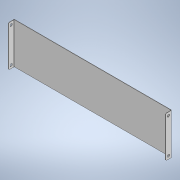
# Autodesk Inventor part: Conector
Saved by Autodesk Inventor 2021.2 (Build 252289000, 289)
## iProperties
Created: 2026-06-03
Part Number: Conector
Material: Generic
Document SubType Name: Sheet Metal
Designer: NELSON
Density: 1 g/cm^3
Sheet Metal Rule: Por defecto_mm
Appearance: Default
Author: NELSON
Autodesk Inventor part; units mm, degrees
ref_plane "YZ Plane" through (0, 0, 0) normal (1, 0, 0) x (0, 1, 0)
ref_plane "XZ Plane" through (0, 0, 0) normal (0, 1, 0) x (-1, 0, 0)
ref_plane "XY Plane" through (0, 0, 0) normal (0, 0, 1) x (1, 0, 0)
sketch "Boceto1" plane through (0, 0, 0) normal (0, 0, 1) x (1, 0, 0)
  line L0 (386.3, -100) -> (-386.3, -100)
  line L1 (-386.3, -100) -> (-386.3, 100)
  line L2 (-386.3, 100) -> (386.3, 100)
  line L3 (386.3, 100) -> (386.3, -100)
  line L4 (386.3, -100) -> (-386.3, 100) construction
  line L5 (-386.3, -100) -> (386.3, 100) construction
  point P0 (0, 0)
  dimension "d0" = 772.6
  dimension "d1" = 200
  measures "d0" distance of L1.end L2.end
  measures "d1" distance of L2.end L0.start
extrude "Placa1" add sketch "Boceto1" along normal blind 2
sketch "Boceto2" plane through (-384.3, -100, 0) normal (-1, 0, 0) x (0, -1, 0)
  line L0 (-200, 0) -> (0, 0)
  line L1 (0, 0) -> (0, 30)
  line L2 (0, 30) -> (-200, 30)
  line L3 (-200, 30) -> (-200, 0)
  constraints: 6 end point, 1 horizontal, 1 perpendicular, 1 vertical
edge flange "Pestaña1" height 30 angle 90 thickness 2 bend radius 2 thickness toward (-1, 0, 0) relief tear relief width 2 relief depth 1 corner gap 2 corner form 0 edges at (-386.3, 0, 2) (386.3, 0, 2) wall of the first edge with corners at (-384.3, 100, 0) (-384.3, -100, 0) (-384.3, -100, 30) (-384.3, 100, 30)
bend "Doblez1"
corner "Esquina1"
sketch "Boceto3" plane through (386.3, -100, 30) normal (1, 0, 0) x (0, 0, -1)
  circle A0 centre (13, 185) radius 6
  circle A1 centre (13, 15) radius 6
  line L0 (26, 0) -> (0, 0) projected
  line L1 (0, 200) -> (26, 200) projected
  point P0 (30, 100)
  point P1 (13, 0)
  point P2 (13, 200)
  dimension "d13" = 12
  dimension "d14" = 12
  dimension "d16" = 15
  dimension "d17" = 15
  constraints: 2 centre point, 2 midpoint, 2 vertical alignment
  measures "d13" diameter of A0
  measures "d14" diameter of A1
  measures "d16" distance from line of L0 A1.centre
  measures "d17" distance from line of A0.centre L1
extrude "Extrusión1" cut sketch "Boceto3" against normal through all
fillet "Redondeo de esquina1" radius 6 4 edges at (385.3, -100, 30) (-385.3, -100, 30) (-385.3, 100, 30) (385.3, 100, 30)
equation "\"d2\" = Thickness"
equation "\"d3\" = BendReliefWidth"
equation "\"d4\" = BendReliefDepth"
equation "\"d5\" = MinimumRemnant"
equation "\"d6\" = TransitionRadius"
equation "\"d9\" = BendRadius"
equation "\"d10\" = CornerReliefSize"
equation "\"d11\" = GapSize"
equation "\"d12\" = JacobiRadiusSize"
equation "\"BendRadius\" = Thickness"
equation "\"BendReliefWidth\" = Thickness"
equation "\"BendReliefDepth\" = 0.5 * Thickness"
equation "\"CornerReliefSize\" = 4 * Thickness"
equation "\"MinimumRemnant\" = 2 * Thickness"
equation "\"TransitionRadius\" = BendRadius"
equation "\"JacobiRadiusSize\" = BendRadius"
equation "\"GapSize\" = Thickness"
equation "\"Thickness\" = 2"
